Autodesk Inventor part; units mm, degrees
(part 2 of 2)
  spline S208 degree 3 poles (-91.9894, 29.864) (-92.0803, 29.584) (-92.1699, 29.3035) (-92.3466, 28.7418) (-92.4337, 28.4606) (-92.5195, 28.1789) knots 0 0 0 0 0.5 0.5 1 1 1 1
  spline S209 degree 3 poles (-95.6824, 33.0065) (-95.1182, 32.426) (-94.5268, 31.8725) (-93.2937, 30.8232) (-92.6527, 30.328) (-91.9894, 29.864) knots 0 0 0 0 0.5 0.5 1 1 1 1
  arc A71 (-95.0636, 34.7486) -> (-95.6824, 33.0065) centre (0, 0) ccw
  spline S210 degree 3 poles (-90.2157, 34.8573) (-91.0231, 34.9157) (-91.8329, 34.9358) (-93.4516, 34.8995) (-94.2596, 34.8431) (-95.0636, 34.7486) knots 0 0 0 0 0.5 0.5 1 1 1 1
  spline S211 degree 3 poles (-89.564, 36.4991) (-89.6751, 36.2265) (-89.785, 35.9533) (-90.0022, 35.406) (-90.1096, 35.1319) (-90.2157, 34.8573) knots 0 0 0 0 0.5 0.5 1 1 1 1
  spline S212 degree 3 poles (-93.0178, 39.9028) (-92.4975, 39.2827) (-91.9481, 38.6875) (-90.7949, 37.551) (-90.1917, 37.0104) (-89.564, 36.4991) knots 0 0 0 0 0.5 0.5 1 1 1 1
  arc A72 (-92.2735, 41.5951) -> (-93.0178, 39.9028) centre (0, 0) ccw
  spline S213 degree 3 poles (-87.4306, 41.3496) (-88.2316, 41.4668) (-89.0378, 41.546) (-90.6548, 41.628) (-91.4648, 41.6307) (-92.2735, 41.5951) knots 0 0 0 0 0.5 0.5 1 1 1 1
  spline S214 degree 3 poles (-86.6608, 42.9395) (-86.7915, 42.6757) (-86.9211, 42.4113) (-87.1777, 41.8813) (-87.3048, 41.6157) (-87.4306, 41.3496) knots 0 0 0 0 0.5 0.5 1 1 1 1
  spline S215 degree 3 poles (-89.857, 46.5863) (-89.3833, 45.9298) (-88.8788, 45.296) (-87.8117, 44.0784) (-87.2496, 43.4952) (-86.6608, 42.9395) knots 0 0 0 0 0.5 0.5 1 1 1 1
  arc A73 (-88.9911, 48.2196) -> (-89.857, 46.5863) centre (0, 0) ccw
  spline S216 degree 3 poles (-84.1791, 47.6213) (-84.9694, 47.7967) (-85.7676, 47.9345) (-87.3743, 48.1343) (-88.1819, 48.1961) (-88.9911, 48.2196) knots 0 0 0 0 0.5 0.5 1 1 1 1
  spline S217 degree 3 poles (-83.2953, 49.1508) (-83.4449, 48.8972) (-83.5934, 48.643) (-83.888, 48.1332) (-84.0341, 47.8776) (-84.1791, 47.6213) knots 0 0 0 0 0.5 0.5 1 1 1 1
  spline S218 degree 3 poles (-86.2167, 53.0211) (-85.7922, 52.3318) (-85.3353, 51.6629) (-84.3599, 50.3707) (-83.8419, 49.748) (-83.2953, 49.1508) knots 0 0 0 0 0.5 0.5 1 1 1 1
  arc A74 (-85.2339, 54.5869) -> (-86.2167, 53.0211) centre (0, 0) ccw
  spline S219 degree 3 poles (-80.4784, 53.6389) (-81.2538, 53.8715) (-82.0398, 54.0673) (-83.6276, 54.3838) (-84.4286, 54.5044) (-85.2339, 54.5869) knots 0 0 0 0 0.5 0.5 1 1 1 1
  spline S220 degree 3 poles (-79.4853, 55.0999) (-79.653, 54.8579) (-79.8196, 54.6152) (-80.1507, 54.1282) (-80.3151, 53.8839) (-80.4784, 53.6389) knots 0 0 0 0 0.5 0.5 1 1 1 1
  spline S221 degree 3 poles (-82.1164, 59.1731) (-81.7433, 58.4546) (-81.3365, 57.7542) (-80.458, 56.3942) (-79.9868, 55.7353) (-79.4853, 55.0999) knots 0 0 0 0 0.5 0.5 1 1 1 1
  arc A75 (-81.0219, 60.663) -> (-82.1164, 59.1731) centre (0, 0) ccw
  spline S222 degree 3 poles (-76.3483, 59.3704) (-77.1047, 59.6589) (-77.8743, 59.9116) (-79.4348, 60.3431) (-80.2248, 60.5219) (-81.0219, 60.663) knots 0 0 0 0 0.5 0.5 1 1 1 1
  spline S223 degree 3 poles (-75.2512, 60.7549) (-75.4361, 60.5258) (-75.6201, 60.2959) (-75.9857, 59.8344) (-76.1675, 59.6028) (-76.3483, 59.3704) knots 0 0 0 0 0.5 0.5 1 1 1 1
  spline S224 degree 3 poles (-77.578, 65.0093) (-77.2584, 64.2656) (-76.9038, 63.5373) (-76.1269, 62.1168) (-75.705, 61.4253) (-75.2512, 60.7549) knots 0 0 0 0 0.5 0.5 1 1 1 1
  arc A76 (-76.3777, 66.4154) -> (-77.578, 65.0093) centre (0, 0) ccw
  spline S225 degree 3 poles (-71.8108, 64.7851) (-72.5441, 65.1281) (-73.2932, 65.4362) (-74.8181, 65.9805) (-75.593, 66.2165) (-76.3777, 66.4154) knots 0 0 0 0 0.5 0.5 1 1 1 1
  spline S226 degree 3 poles (-70.6156, 66.0858) (-70.8168, 65.8709) (-71.017, 65.655) (-71.4154, 65.2214) (-71.6136, 65.0037) (-71.8108, 64.7851) knots 0 0 0 0 0.5 0.5 1 1 1 1
  spline S227 degree 3 poles (-72.6256, 70.4987) (-72.3612, 69.7336) (-72.0607, 68.9814) (-71.3895, 67.508) (-71.0193, 66.7875) (-70.6156, 66.0858) knots 0 0 0 0 0.5 0.5 1 1 1 1
  arc A77 (-71.3259, 71.8134) -> (-72.6256, 70.4987) centre (0, 0) ccw
  spline S228 degree 3 poles (-66.8903, 69.8541) (-67.5966, 70.2497) (-68.3212, 70.6117) (-69.8022, 71.2659) (-70.5578, 71.5578) (-71.3259, 71.8134) knots 0 0 0 0 0.5 0.5 1 1 1 1
  spline S229 degree 3 poles (-65.6033, 71.0641) (-65.8196, 70.8644) (-66.035, 70.6637) (-66.464, 70.2604) (-66.6776, 70.0577) (-66.8903, 69.8541) knots 0 0 0 0 0.5 0.5 1 1 1 1
  spline S230 degree 3 poles (-67.2858, 75.612) (-67.0779, 74.8296) (-66.8331, 74.0575) (-66.2713, 72.539) (-65.9547, 71.7934) (-65.6033, 71.0641) knots 0 0 0 0 0.5 0.5 1 1 1 1
  arc A78 (-65.8936, 76.8283) -> (-67.2858, 75.612) centre (0, 0) ccw
  spline S231 degree 3 poles (-61.6128, 74.5504) (-62.2883, 74.9965) (-62.9846, 75.4104) (-64.4139, 76.171) (-65.1462, 76.5173) (-65.8936, 76.8283) knots 0 0 0 0 0.5 0.5 1 1 1 1
  spline S232 degree 3 poles (-60.2409, 75.6633) (-60.4713, 75.4799) (-60.7008, 75.2955) (-61.1581, 74.9245) (-61.3859, 74.738) (-61.6128, 74.5504) knots 0 0 0 0 0.5 0.5 1 1 1 1
  spline S233 degree 3 poles (-61.587, 80.3218) (-61.4368, 79.5264) (-61.249, 78.7384) (-60.7995, 77.183) (-60.5381, 76.4163) (-60.2409, 75.6633) knots 0 0 0 0 0.5 0.5 1 1 1 1
  arc A79 (-60.1097, 81.4333) -> (-61.587, 80.3218) centre (0, 0) ccw
  spline S234 degree 3 poles (-56.0066, 78.849) (-56.6478, 79.3432) (-57.312, 79.8068) (-58.682, 80.6697) (-59.387, 81.0685) (-60.1097, 81.4333) knots 0 0 0 0 0.5 0.5 1 1 1 1
  spline S235 degree 3 poles (-54.5572, 79.8587) (-54.8003, 79.6927) (-55.0426, 79.5255) (-55.5258, 79.1889) (-55.7666, 79.0195) (-56.0066, 78.849) knots 0 0 0 0 0.5 0.5 1 1 1 1
  spline S236 degree 3 poles (-55.5596, 84.6031) (-55.4678, 83.7988) (-55.338, 82.9993) (-55.0033, 81.4151) (-54.7986, 80.6314) (-54.5572, 79.8587) knots 0 0 0 0 0.5 0.5 1 1 1 1
  arc A80 (-54.0051, 85.6038) -> (-55.5596, 84.6031) centre (0, 0) ccw
  spline S237 degree 3 poles (-50.1016, 82.7269) (-50.705, 83.2666) (-51.3336, 83.7774) (-52.6369, 84.738) (-53.311, 85.1872) (-54.0051, 85.6038) knots 0 0 0 0 0.5 0.5 1 1 1 1
  spline S238 degree 3 poles (-48.5823, 83.6281) (-48.8369, 83.4802) (-49.0908, 83.3312) (-49.5972, 83.0308) (-49.8497, 82.8794) (-50.1016, 82.7269) knots 0 0 0 0 0.5 0.5 1 1 1 1
  spline S239 degree 3 poles (-49.2357, 88.433) (-49.2029, 87.6241) (-49.1319, 86.8173) (-48.9137, 85.2129) (-48.7667, 84.4164) (-48.5823, 83.6281) knots 0 0 0 0 0.5 0.5 1 1 1 1
  arc A81 (-47.6124, 89.3175) -> (-49.2357, 88.433) centre (0, 0) ccw
  spline S240 degree 3 poles (-43.9293, 86.1634) (-44.4916, 86.7457) (-45.0812, 87.3011) (-46.311, 88.3542) (-46.9505, 88.8514) (-47.6124, 89.3175) knots 0 0 0 0 0.5 0.5 1 1 1 1
  spline S241 degree 3 poles (-42.3482, 86.9513) (-42.6129, 86.8224) (-42.877, 86.6923) (-43.4041, 86.4296) (-43.667, 86.2971) (-43.9293, 86.1634) knots 0 0 0 0 0.5 0.5 1 1 1 1
  spline S242 degree 3 poles (-42.6492, 91.7911) (-42.6755, 90.982) (-42.6635, 90.1721) (-42.563, 88.5561) (-42.4746, 87.7509) (-42.3482, 86.9513) knots 0 0 0 0 0.5 0.5 1 1 1 1
  arc A82 (-40.9656, 92.5547) -> (-42.6492, 91.7911) centre (0, 0) ccw
  spline S243 degree 3 poles (-37.5225, 89.1401) (-38.0409, 89.7619) (-38.5884, 90.3589) (-39.738, 91.499) (-40.3395, 92.0415) (-40.9656, 92.5547) knots 0 0 0 0 0.5 0.5 1 1 1 1
  spline S244 degree 3 poles (-35.8882, 89.8106) (-36.1616, 89.7013) (-36.4345, 89.5908) (-36.9793, 89.3673) (-37.2512, 89.2543) (-37.5225, 89.1401) knots 0 0 0 0 0.5 0.5 1 1 1 1
  spline S245 degree 3 poles (-35.8351, 94.6594) (-35.9204, 93.8544) (-35.9676, 93.0457) (-35.9853, 91.4267) (-35.9559, 90.6173) (-35.8882, 89.8106) knots 0 0 0 0 0.5 0.5 1 1 1 1
  arc A83 (-34.1002, 95.2981) -> (-35.8351, 94.6594) centre (0, 0) ccw
  circle A84 centre (-70.2676, -40.7925) radius 5.4821
  circle A85 centre (70.4611, -40.4572) radius 5.4821
  circle A86 centre (-0.1936, 81.2498) radius 5.4821
  circle A87 centre (70.2676, 40.7925) radius 5.4821
  circle A88 centre (0.1936, -81.2498) radius 5.4821
  circle A89 centre (-70.4611, 40.4572) radius 5.4821
  spline S246 degree 3 poles (-10.2504, 96.1708) (-10.5677, 96.9156) (-10.92, 97.645) (-11.6924, 99.068) (-12.112, 99.7608) (-12.5637, 100.4326) knots 0 0 0 0 0.5 0.5 1 1 1 1
  spline S247 degree 3 poles (-7.0444, 100.97) (-7.358, 100.2236) (-7.6362, 99.4629) (-8.1196, 97.9176) (-8.3246, 97.134) (-8.4922, 96.342) knots 0 0 0 0 0.5 0.5 1 1 1 1
  spline S248 degree 3 poles (-3.2031, 96.6625) (-3.4651, 97.4285) (-3.7632, 98.1816) (-4.4297, 99.6572) (-4.7977, 100.3788) (-5.1991, 101.0818) knots 0 0 0 0 0.5 0.5 1 1 1 1
  spline S249 degree 3 poles (-14.3959, 100.1864) (-14.6543, 99.4192) (-14.8761, 98.6401) (-15.2455, 97.0637) (-15.3927, 96.2672) (-15.5021, 95.4651) knots 0 0 0 0 0.5 0.5 1 1 1 1
  arc A90 (-5.1991, 101.0818) -> (-7.0444, 100.97) centre (0, 0) ccw
  spline S250 degree 3 poles (-30.9156, 91.6413) (-31.3872, 92.2993) (-31.8897, 92.9346) (-32.953, 94.1556) (-33.5133, 94.7406) (-34.1002, 95.2981) knots 0 0 0 0 0.5 0.5 1 1 1 1
  spline S251 degree 3 poles (-29.2367, 92.1907) (-29.5174, 92.1016) (-29.7976, 92.0114) (-30.3573, 91.8282) (-30.6367, 91.7354) (-30.9156, 91.6413) knots 0 0 0 0 0.5 0.5 1 1 1 1
  spline S252 degree 3 poles (-28.8298, 97.0227) (-28.9736, 96.226) (-29.0797, 95.423) (-29.2156, 93.8096) (-29.2453, 93.0002) (-29.2367, 92.1907) knots 0 0 0 0 0.5 0.5 1 1 1 1
  arc A91 (-27.053, 97.533) -> (-28.8298, 97.0227) centre (0, 0) ccw
  spline S253 degree 3 poles (-24.1438, 93.6535) (-24.5661, 94.3442) (-25.0208, 95.0145) (-25.9922, 96.3098) (-26.5082, 96.9342) (-27.053, 97.533) knots 0 0 0 0 0.5 0.5 1 1 1 1
  spline S254 degree 3 poles (-22.4293, 94.0789) (-22.7156, 94.0106) (-23.0017, 93.941) (-23.5732, 93.7992) (-23.8587, 93.727) (-24.1438, 93.6535) knots 0 0 0 0 0.5 0.5 1 1 1 1
  spline S255 degree 3 poles (-21.6707, 98.8683) (-21.8723, 98.0842) (-22.0367, 97.2911) (-22.29, 95.6919) (-22.3787, 94.8868) (-22.4293, 94.0789) knots 0 0 0 0 0.5 0.5 1 1 1 1
  arc A92 (-19.8613, 99.2476) -> (-21.6707, 98.8683) centre (0, 0) ccw
  spline S256 degree 3 poles (-17.2431, 95.1661) (-17.6139, 95.8857) (-18.0185, 96.5874) (-18.8927, 97.9502) (-19.3618, 98.6105) (-19.8613, 99.2476) knots 0 0 0 0 0.5 0.5 1 1 1 1
  spline S257 degree 3 poles (-15.5021, 95.4651) (-15.7927, 95.4179) (-16.0831, 95.3694) (-16.6635, 95.2697) (-16.9534, 95.2185) (-17.2431, 95.1661) knots 0 0 0 0 0.5 0.5 1 1 1 1
  point P0 (0, 0)
  point P1 (0, 0)
  point P2 (0, 0)
  point P3 (0, 0)
  point P4 (0, 0)
extrude "Выдавливание3" [suppressed]
sketch "Эскиз5" plane through (0, 0, 10) normal (0, 0, 1) x (1, 0, 0)
  circle A0 centre (0, 0) radius 67.5 projected
  circle A1 centre (0, 0) radius 96.7017
  circle A2 centre (0, 0) radius 81.25
  circle A3 centre (0, -81.25) radius 2.15
  circle A4 centre (70.3646, -40.625) radius 2.15
  circle A5 centre (70.3646, 40.625) radius 2.15
  circle A6 centre (0, 81.25) radius 2.15
  circle A7 centre (-70.3646, 40.625) radius 2.15
  circle A8 centre (-70.3646, -40.625) radius 2.15
  dimension "d54" = 162.5
  dimension "d55" = 4.3
  dimension "d58" = 360
  constraints: 7 centre point, 2 coincident, 1 vertical alignment, 15 other
  measures "d55" diameter of A3
extrude "Выдавливание4" cut sketch "Эскиз5" against normal through all contours A5 A2 | A2 A5 | A4 A2 | A2 A4 | A6 A2 | A2 A6 | A3 A2 | A2 A3 | A7 A2 | A2 A7 | A8 A2 | A2 A8
equation "\"d0\" = da_da"
equation "\"d1\" = da_b"
equation "\"d3\" = da_d"
equation "\"da_da\" = 202.430781"
equation "\"da_b\" = 10"
equation "\"da_d\" = 198.608493"
body "Solid1"
body "Srf1"
